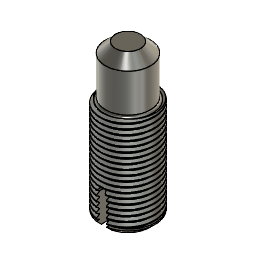
Screw (Autodesk Fusion 360 design; units mm, degrees)
Autodesk Fusion 360 part; units mm, degrees
sketch "Sketch1" plane through (0, 0, 0) normal (0, 0, 1) x (1, 0, 0)
  circle A0 centre (0, 0) radius 2.7
  line L0 (-0.5, 2.6533) -> (-0.5, -2.6533)
  line L1 (0, 0) -> (0, 2.7) construction
  line L2 (0.5, 2.6533) -> (0.5, -2.6533)
  dimension "d1" = 5.4
  dimension "d4" = 0.5
  constraint coincident A0.centre L1.start
  constraint coincident A0 L0.start
  constraint coincident A0 L0.end
  constraint vertical L0
  constraint coincident A0 L1.end
  constraint parallel L0 L1
  constraint symmetric L0.start L1 L2.start
  constraint symmetric L0.end L1 L2.end
  measures "d1" diameter of A0
  measures "d4" distance of L0 L1
extrude "Extrude1" add sketch "Sketch1" along normal blind 10
extrude "Extrude2" cut sketch "Sketch1" along normal blind 3.5 contours A0 L0 L2
sketch "Sketch2" plane through (0, 0, 10) normal (0, 0, 1) x (-1, 0, 0)
  circle A0 centre (0, 0) radius 2.7
  circle A1 centre (0, 0) radius 2.25
  dimension "d12" = 4.5
  constraint coincident A0.centre A1.centre
  measures "d12" diameter of A1
extrude "Extrude3" add sketch "Sketch2" along normal blind 5 contours A1
chamfer "Chamfer2" distance 1 angle 45 1 edges at (2.0977, 0.8136, 15)
chamfer "Chamfer4" distance 0.5 angle 45 2 edges at (-2.7, 0, 0) (2.7, 0, 0)
fillet "Fillet3" radius 0.5 2 edges at (-0.5, 0, 3.5) (0.5, 0, 3.5)
thread "Thread2" "ISO Metric profile 5.5 M5.5x0.5 M5.5x0.5 6g" major diameter 5.427 minor diameter 4.848 pitch 0.5 angle 60 modelled right hand crest width 0.0671 on face at (-0.7912, -2.5815, 4.5) crest through (2.7135, 0, 0.375)
fillet "Fillet4" radius 0.2 1 edges at (2.0977, -0.8136, 10)
